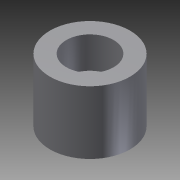
# Autodesk Inventor part: Screw_Asm_Jig_Lower
Saved by Autodesk Inventor 2011 SP2 (Build 150309200, 309)
## iProperties
Created: 2012-02-15
Part Number: Screw_Asm_Jig_Lower
Document SubType Name: Modeling
Designer: sungwook
Density: 1 g/cm^3
Author: sungwook
Autodesk Inventor part; units mm, degrees
ref_plane "YZ Plane" through (0, 0, 0) normal (1, 0, 0) x (0, 1, 0)
ref_plane "XZ Plane" through (0, 0, 0) normal (0, 1, 0) x (-1, 0, 0)
ref_plane "XY Plane" through (0, 0, 0) normal (0, 0, 1) x (1, 0, 0)
sketch "Sketch1" plane through (0, 0, 0) normal (0, 0, 1) x (1, 0, 0)
  circle A0 centre (0, 0) radius 12.7
  dimension "d0" = 25.4
  constraints: 1 centre point, 1 coincident
  measures "d0" diameter of A0
extrude "Extrusion1" add sketch "Sketch1" along normal blind 10
hole "Hole1" at (0, 0, 10) direction (0, 0, -1) diameter 2.4 depth 2
hole "Hole2" at (0, 0, 8) direction (0, 0, -1) diameter 2 end through all
sketch "Sketch2" plane through (0, 0, 10) normal (0, 0, 1) x (1, 0, 0)
  circle A0 centre (0, 0) radius 12.7 projected
  circle A1 centre (0, 0) radius 7.5
  dimension "d21" = 15
  constraints: 1 centre point, 1 coincident
  measures "d21" diameter of A1
extrude "Extrusion2" add sketch "Sketch2" along normal blind 10
body "Solid1"
